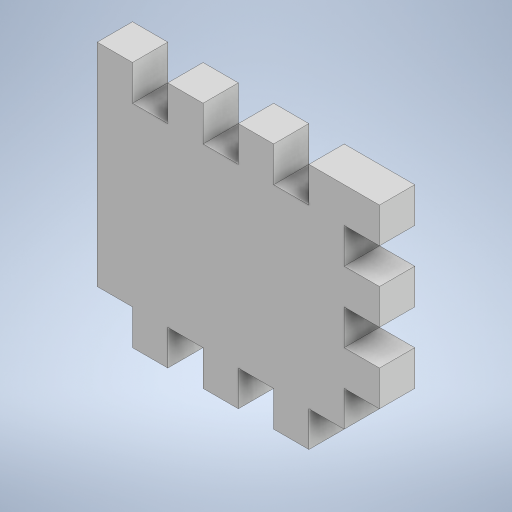
# Autodesk Inventor part: backside
Saved by Autodesk Inventor 2024 (Build 280153000, 153)
## iProperties
Created: 2024-04-15
Part Number: backside
Material: Generic
Document SubType Name: Modeling
Designer: srika
Density: 1 g/cm^3
Appearance: Default
Author: srika
Autodesk Inventor part; units mm, degrees
ref_plane "YZ Plane" through (0, 0, 0) normal (1, 0, 0) x (0, 1, 0)
ref_plane "XZ Plane" through (0, 0, 0) normal (0, 1, 0) x (-1, 0, 0)
ref_plane "XY Plane" through (0, 0, 0) normal (0, 0, 1) x (1, 0, 0)
sketch "Sketch2" plane through (0, 0, 0) normal (0, 0, 1) x (1, 0, 0)
  line L0 (5, 5) -> (10, 5)
  line L1 (10, 5) -> (10, 0)
  line L2 (10, 0) -> (5, 0)
  line L3 (5, 0) -> (5, 5)
  line L4 (0, 5) -> (40, 5)
  line L5 (40, 5) -> (40, 30)
  line L6 (40, 30) -> (0, 30)
  line L7 (0, 30) -> (0, 5)
  line L8 (20, 5) -> (20, 0)
  line L9 (20, 0) -> (15, 0)
  line L10 (15, 0) -> (15, 5)
  line L11 (30, 5) -> (30, 0)
  line L12 (30, 0) -> (25, 0)
  line L13 (25, 0) -> (25, 5)
  line L14 (40, 20) -> (40, 15)
  line L15 (40, 10) -> (40, 5)
  line L16 (40, 30) -> (40, 5)
  line L17 (35, 25) -> (40, 25)
  line L18 (40, 25) -> (40, 20)
  line L19 (40, 20) -> (35, 20)
  line L20 (35, 20) -> (35, 25)
  line L21 (35, 15) -> (40, 15)
  line L22 (40, 15) -> (40, 10)
  line L23 (40, 10) -> (35, 10)
  line L24 (35, 10) -> (35, 15)
  line L25 (10, 30) -> (5, 30)
  line L26 (20, 30) -> (15, 30)
  line L27 (30, 30) -> (25, 30)
  line L28 (40, 30) -> (35, 30)
  line L29 (0, 35) -> (5, 35)
  line L30 (5, 35) -> (5, 30)
  line L31 (5, 30) -> (0, 30)
  line L32 (0, 30) -> (0, 35)
  line L33 (15, 35) -> (15, 30)
  line L34 (15, 30) -> (10, 30)
  line L35 (10, 30) -> (10, 35)
  line L36 (10, 35) -> (15, 35)
  line L37 (25, 35) -> (25, 30)
  line L38 (25, 30) -> (20, 30)
  line L39 (20, 30) -> (20, 35)
  line L40 (20, 35) -> (25, 35)
  line L41 (35, 35) -> (35, 30)
  line L42 (35, 30) -> (30, 30)
  line L43 (30, 30) -> (30, 35)
  line L44 (30, 35) -> (35, 35)
  line L45 (40, 0) -> (35, 0)
  line L46 (35, 0) -> (35, 35)
  line L47 (35, 35) -> (40, 35)
  line L48 (40, 35) -> (40, 0)
  point P0 (0, 0)
  point P1 (35, 5)
  dimension "d105" = 10
  dimension "d110" = 40
  dimension "d115" = 10
  constraints: 98 end point, 12 parallel, 8 horizontal, 6 perpendicular, 4 point on line, 1 midpoint, 41 other
  measures "d105" distance of L1.end L8.end
  measures "d110" distance of L5.end L6.end
  measures "d115" distance of L6.end point (10, 30)
extrude "Extrusion3" add sketch "Sketch2" along normal blind 5 contours L4 L7 L6 L46 L20 L24 L0 | L0 L1 L2 L3 | L4 L8 L9 L10 | L32 L29 L30 L6 | L4 L11 L12 L13 | L35 L36 L33 L6 | L39 L40 L37 L6 | L24 L21 L5 L23 | L43 L44 L41 L6 | L20 L17 L5 L19 | L41 L47 L48 L6
body "Solid3"
